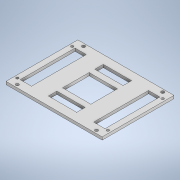
# Autodesk Inventor part: reg_board_plate
Saved by Autodesk Inventor 2020 (Build 240168000, 168)
## iProperties
Created: 2022-10-27
Part Number: reg_board_plate
Material: 일반
Document SubType Name: Modeling
Designer: SeungJin
Density: 1 g/cm^3
Appearance: 기본값
Author: SeungJin
Autodesk Inventor part; units mm, degrees
ref_plane "YZ Plane" through (0, 0, 0) normal (1, 0, 0) x (0, 1, 0)
ref_plane "XZ Plane" through (0, 0, 0) normal (0, 1, 0) x (-1, 0, 0)
ref_plane "XY Plane" through (0, 0, 0) normal (0, 0, 1) x (1, 0, 0)
sketch "스케치1" plane through (0, 0, 0) normal (0, 1, 0) x (-1, 0, 0)
  line L0 (70, 58.5) -> (-70, 58.5)
  line L1 (-70, 58.5) -> (-70, -58.5)
  line L2 (-70, -58.5) -> (70, -58.5)
  line L3 (70, -58.5) -> (70, 58.5)
  line L4 (70, 58.5) -> (-70, -58.5) construction
  line L5 (-70, 58.5) -> (70, -58.5) construction
  line L6 (85, -63.5) -> (-85, -63.5)
  line L7 (-85, -63.5) -> (-85, 63.5)
  line L8 (-85, 63.5) -> (85, 63.5)
  line L9 (85, 63.5) -> (85, -63.5)
  line L10 (85, -63.5) -> (-85, 63.5) construction
  line L11 (-85, -63.5) -> (85, 63.5) construction
  point P0 (0, 0)
  dimension "d0" = 140
  dimension "d1" = 117
  dimension "d2" = 170
  dimension "d3" = 127
  constraints: 24 end point, 4 midpoint, 4 parallel, 2 horizontal, 2 perpendicular
  measures "d0" distance of L2.end L1.end
  measures "d1" distance of L1.end L0.end
  measures "d2" distance of L7.end L8.end
  measures "d3" distance of L6.end L7.end
extrude "돌출1" add sketch "스케치1" along normal blind 5 contours L3 L2 L1 L0 | L6 L7 L8 L9
sketch "스케치2" plane through (0, 0, 0) normal (0, -1, 0) x (1, 0, 0)
  line L0 (-70, 58.5) -> (70, 58.5)
  line L1 (70, 58.5) -> (70, -58.5)
  line L2 (70, -58.5) -> (-70, -58.5)
  line L3 (-70, -58.5) -> (-70, 58.5)
  line L4 (-70, 58.5) -> (70, -58.5) construction
  line L5 (70, 58.5) -> (-70, -58.5) construction
  point P0 (0, 0)
  dimension "d6" = 140
  dimension "d7" = 117
  constraints: 12 end point, 2 midpoint, 2 parallel, 1 horizontal, 1 perpendicular
  measures "d6" distance of L1.end L2.end
  measures "d7" distance of L0.end L1.end
hole "구멍1" at (-70, 0, 58.5) at (70, 0, 58.5) at (-70, 0, -58.5) at (70, 0, -58.5) direction (0, 1, 0) diameter 5.5 end through all clearance for "Socket Head Cap Screw ISO 4762" size "M5" standard "ISO"
sketch "스케치3" plane through (0, 0, 0) normal (0, -1, 0) x (1, 0, 0)
  line L0 (-85, -63.5) -> (-85, 63.5) projected
  line L1 (85, 63.5) -> (85, -63.5) projected
  line L2 (85, -63.5) -> (-85, -63.5) projected
  line L3 (-85, 63.5) -> (85, 63.5) projected
  line L4 (-55, 48.5) -> (-55, -48.5)
  line L5 (85, -63.5) -> (-85, -63.5) projected
  line L6 (55, 48.5) -> (55, -48.5)
  line L7 (-25, 33.5) -> (25, 33.5)
  line L8 (-25, 23.5) -> (25, 23.5)
  line L9 (-25, -23.5) -> (25, -23.5)
  line L10 (-25, -33.5) -> (25, -33.5)
  line L11 (55, 48.5) -> (75, 48.5)
  line L12 (-75, 48.5) -> (-55, 48.5)
  line L13 (-25, 48.5) -> (25, 48.5)
  line L14 (-75, -48.5) -> (-55, -48.5)
  line L15 (-25, -48.5) -> (25, -48.5)
  line L16 (55, -48.5) -> (75, -48.5)
  line L17 (25, -33.5) -> (25, -48.5)
  line L18 (-25, -33.5) -> (-25, -48.5)
  line L19 (-25, 48.5) -> (-25, 33.5)
  line L20 (-25, 23.5) -> (-25, -23.5)
  line L21 (25, 48.5) -> (25, 33.5)
  line L22 (25, 23.5) -> (25, -23.5)
  line L23 (-75, -48.5) -> (-75, 48.5)
  line L24 (75, -48.5) -> (75, 48.5)
  point P0 (0, 0)
  point P1 (-75, -48.5)
  dimension "d24" = 10
  dimension "d26" = 10
  dimension "d28" = 15
  dimension "d29" = 15
  dimension "d30" = 15
  dimension "d31" = 15
  dimension "d32" = 15
  dimension "d33" = 15
  dimension "d34" = 15
  dimension "d35" = 15
  dimension "d36" = 30
  dimension "d37" = 30
  dimension "d38" = 30
  dimension "d39" = 30
  dimension "d40" = 30
  dimension "d41" = 30
  dimension "d44" = 10
  dimension "d45" = 10
  dimension "d46" = 20
  dimension "d47" = 20
  constraints: 40 end point, 13 perpendicular, 3 horizontal, 1 parallel
  measures "d24" distance between parallel lines of L7 L8
  measures "d26" distance between parallel lines of L9 L10
  measures "d28" distance between parallel lines of L2 L15
  measures "d29" distance between parallel lines of L7 L13
  measures "d30" distance between parallel lines of L15 L10
  measures "d31" distance between parallel lines of L3 L13
  measures "d32" distance between parallel lines of L3 L11
  measures "d33" distance between parallel lines of L3 L12
  measures "d34" distance between parallel lines of L5 L14
  measures "d35" distance between parallel lines of L2 L16
  measures "d36" distance between parallel lines of L6 L21
  measures "d37" distance between parallel lines of L22 L6
  measures "d38" distance between parallel lines of L17 L6
  measures "d39" distance between parallel lines of L4 L18
  measures "d40" distance between parallel lines of L4 L20
  measures "d41" distance between parallel lines of L4 L19
  measures "d44" distance between parallel lines of L0 L23
  measures "d45" distance between parallel lines of L24 L1
  measures "d46" distance between parallel lines of L4 L23
  measures "d47" distance between parallel lines of L24 L6
extrude "돌출2" cut sketch "스케치3" against normal blind 5 contours L4 L14 L23 L12 | L11 L24 L16 L6 | L19 L13 L21 L7 | L8 L22 L9 L20 | L10 L17 L15 L18
sketch "스케치4" plane through (0, 0, 0) normal (0, -1, 0) x (1, 0, 0)
  line L0 (-25, -48.5) -> (-25, -33.5) projected
  line L1 (-25, -33.5) -> (25, -33.5) projected
  line L2 (25, -33.5) -> (25, -48.5) projected
  line L3 (25, -48.5) -> (-25, -48.5) projected
  line L4 (25, 33.5) -> (-25, 33.5) projected
  line L5 (-25, 33.5) -> (-25, 48.5) projected
  line L6 (-25, 48.5) -> (25, 48.5) projected
  line L7 (25, 48.5) -> (25, 33.5) projected
  line L8 (25, 23.5) -> (25, -23.5) projected
  line L9 (25, -23.5) -> (-25, -23.5) projected
  line L10 (-25, -23.5) -> (-25, 23.5) projected
  line L11 (-25, 23.5) -> (25, 23.5) projected
  line L12 (55, 48.5) -> (75, 48.5) projected
  line L13 (75, 48.5) -> (75, -48.5) projected
  line L14 (75, -48.5) -> (55, -48.5) projected
  line L15 (55, -48.5) -> (55, 48.5) projected
  line L16 (-55, -48.5) -> (-75, -48.5) projected
  line L17 (-75, -48.5) -> (-75, 48.5) projected
  line L18 (-75, 48.5) -> (-55, 48.5) projected
  line L19 (-55, 48.5) -> (-55, -48.5) projected
  circle A0 centre (-70, -58.5) radius 2.75 projected
  circle A1 centre (-70, 58.5) radius 2.75 projected
  circle A2 centre (70, 58.5) radius 2.75 projected
  circle A3 centre (70, -58.5) radius 2.75 projected
  line L20 (85, 63.5) -> (85, -63.5) projected
  line L21 (-85, 63.5) -> (85, 63.5) projected
  line L22 (-85, -63.5) -> (-85, 63.5) projected
  line L23 (85, -63.5) -> (-85, -63.5) projected
  line L24 (-80, -48.5) -> (80, -48.5)
  line L25 (80, -48.5) -> (80, 48.5)
  line L26 (80, 48.5) -> (-80, 48.5)
  line L27 (-80, 48.5) -> (-80, -48.5)
  line L28 (-80, -48.5) -> (80, 48.5) construction
  line L29 (80, -48.5) -> (-80, 48.5) construction
  point P0 (0, 0)
  dimension "d48" = 160
  dimension "d49" = 97
  constraints: 12 end point, 2 midpoint, 2 parallel, 1 horizontal, 1 perpendicular
  measures "d48" distance of L26.end L25.end
  measures "d49" distance of L24.end L25.end
hole "구멍2" at (-80, 0, 48.5) at (80, 0, 48.5) at (80, 0, -48.5) at (-80, 0, -48.5) direction (0, 1, 0) diameter 4.5 end through all clearance for "Socket Head Cap Screw ISO 4762" size "M4" standard "ISO"
